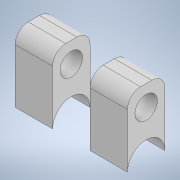
# Autodesk Inventor part: harness attachments
Saved by Autodesk Inventor 2021 (Build 250183000, 183)
## iProperties
Created: 2020-10-11
Part Number: harness attachments
Material: Generic
Document SubType Name: Modeling
Designer: atwaterh
Density: 1 g/cm^3
Appearance: Default
Author: atwaterh
Autodesk Inventor part; units mm, degrees
ref_plane "YZ Plane" through (0, 0, 0) normal (1, 0, 0) x (0, 1, 0)
ref_plane "XZ Plane" through (0, 0, 0) normal (0, 1, 0) x (-1, 0, 0)
ref_plane "XY Plane" through (0, 0, 0) normal (0, 0, 1) x (1, 0, 0)
sketch "Sketch1" plane through (0, 0, 0) normal (1, 0, 0) x (0, 1, 0)
  line L0 (13.97, 12.7) -> (-22.86, 12.7)
  line L1 (-22.86, -12.7) -> (13.97, -12.7)
  line L2 (22.86, -3.81) -> (22.86, 3.81)
  line L3 (22.86, 12.7) -> (-22.86, -12.7) construction
  line L4 (-22.86, 12.7) -> (22.86, -12.7) construction
  circle A0 centre (8.89, 0) radius 7.62
  arc A1 (22.86, 3.81) -> (13.97, 12.7) centre (13.97, 3.81) ccw
  arc A2 (13.97, -12.7) -> (22.86, -3.81) centre (13.97, -3.81) ccw
  arc A3 (-22.86, -12.7) -> (-22.86, 12.7) centre (-22.86, 0) ccw
  point P0 (0, 0)
  dimension "d1" = 25.4
  dimension "d2" = 15.24
  dimension "d3" = 8.89
  dimension "d5" = 12.7
  dimension "d6" = 45.72
  dimension "d7" = 31.75
  constraints: 10 end point, 6 point on circle, 4 centre point, 4 point on line, 4 tangent, 2 midpoint, 1 equal radius, 1 horizontal, 1 parallel
  measures "d1" distance of L1.start L0.end
  measures "d2" diameter of A0
  measures "d3" radius of A1
  measures "d5" radius of A3
  measures "d6" distance from line of A3.centre L2
  measures "d7" distance of A3.centre A0.centre
extrude "Extrusion1" add sketch "Sketch1" along normal blind 76.2
sketch "Sketch2" plane through (0, -22.86, 12.7) normal (0, 0, 1) x (1, 0, 0)
  line L0 (0, 0) -> (76.2, 0) projected
  line L1 (25.4034, 0) -> (50.8034, 0)
  line L2 (50.8034, 0) -> (50.8034, 76.2)
  line L3 (50.8034, 76.2) -> (25.4034, 76.2)
  line L4 (25.4034, 76.2) -> (25.4034, 0)
  point P0 (0, 22.86)
  dimension "d10" = 25.4
  dimension "d11" = 76.2
  constraints: 8 end point, 2 parallel, 1 horizontal, 1 perpendicular, 1 point on line
  measures "d10" distance of L3.end L2.end
  measures "d11" distance between parallel lines of L3 L0
extrude "Extrusion2" cut sketch "Sketch2" against normal blind 76.2
equation "\"d12\" = d11"
body "Solid1"
